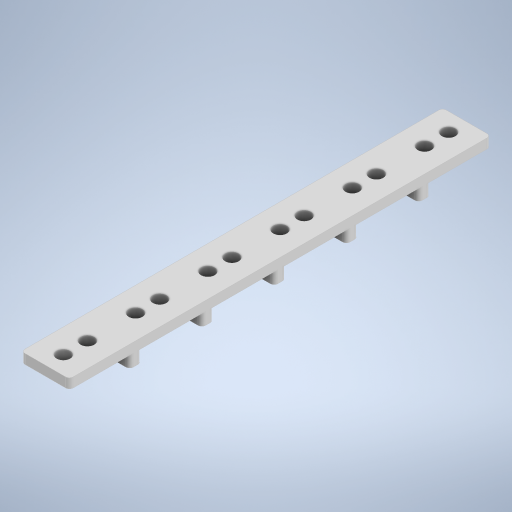
# Autodesk Inventor part: belka_poprzeg
Saved by Autodesk Inventor 2024.2 (Build 282272000, 272)
## iProperties
Created: 2024-01-12
Part Number: belka_poprzeg
Material: PLA
Document SubType Name: Modeling
Designer: Konrad
Density: 1 g/cm^3
Appearance: PLA
Author: Konrad
Autodesk Inventor part; units mm, degrees
ref_plane "YZ Plane" through (0, 0, 0) normal (1, 0, 0) x (0, 1, 0)
ref_plane "XZ Plane" through (0, 0, 0) normal (0, 1, 0) x (-1, 0, 0)
ref_plane "XY Plane" through (0, 0, 0) normal (0, 0, 1) x (1, 0, 0)
sketch "Szkic1" plane through (0, 0, 0) normal (0, 1, 0) x (-1, 0, 0)
  line L0 (0, 0) -> (20, 0)
  line L1 (20, 0) -> (20, -25)
  line L2 (20, -25) -> (0, -25)
  line L3 (0, -25) -> (0, 0)
  line L4 (0, -25) -> (20, -25)
  line L5 (20, -25) -> (20, -30)
  line L6 (20, -30) -> (0, -30)
  line L7 (0, -30) -> (0, -25)
  line L8 (0, -30) -> (20, -30)
  line L9 (0, -30) -> (20, -30)
  line L10 (20, -30) -> (20, -55)
  line L11 (20, -55) -> (0, -55)
  line L12 (0, -55) -> (0, -30)
  line L13 (0, -55) -> (20, -55)
  line L14 (20, -55) -> (20, -60)
  line L15 (20, -60) -> (0, -60)
  line L16 (0, -60) -> (0, -55)
  line L17 (0, -60) -> (12.1994, -60)
  line L18 (0, -60) -> (20, -60)
  line L19 (20, -60) -> (20, -85)
  line L20 (20, -85) -> (0, -85)
  line L21 (0, -85) -> (0, -60)
  line L22 (0, -85) -> (20, -85)
  line L23 (20, -85) -> (20, -90)
  line L24 (20, -90) -> (0, -90)
  line L25 (0, -90) -> (0, -85)
  line L26 (0, -90) -> (12.1994, -90)
  line L27 (0, -90) -> (20, -90)
  line L28 (20, -90) -> (20, -115)
  line L29 (20, -115) -> (0, -115)
  line L30 (0, -115) -> (0, -90)
  line L31 (0, -115) -> (20, -115)
  line L32 (20, -115) -> (20, -120)
  line L33 (20, -120) -> (0, -120)
  line L34 (0, -120) -> (0, -115)
  line L35 (0, -120) -> (3.8166, -120)
  line L36 (20, -120) -> (0, -120)
  line L37 (0, -120) -> (0, -145)
  line L38 (0, -145) -> (20, -145)
  line L39 (20, -145) -> (20, -120)
  circle A0 centre (10, -7.5) radius 2.8
  circle A1 centre (10, -17.5) radius 2.8
  line L40 (20, -42.5) -> (0, -42.5) construction
  line L41 (20, -72.5) -> (0, -72.5) construction
  line L42 (20, -102.5) -> (0, -102.5) construction
  line L43 (20, -132.5) -> (0, -132.5) construction
  line L44 (20, -12.5) -> (0, -12.5) construction
  circle A2 centre (10, -47.5) radius 2.8
  circle A3 centre (10, -37.5) radius 2.8
  circle A4 centre (10, -77.5) radius 2.8
  circle A5 centre (10, -67.5) radius 2.8
  circle A6 centre (10, -107.5) radius 2.8
  circle A7 centre (10, -97.5) radius 2.8
  circle A8 centre (10, -137.5) radius 2.8
  circle A9 centre (10, -127.5) radius 2.8
  circle A10 centre (10, -167.5) radius 2.8
  circle A11 centre (10, -157.5) radius 2.8
  line L45 (20, -145) -> (0, -145)
  line L46 (0, -145) -> (0, -150)
  line L47 (0, -150) -> (20, -150)
  line L48 (20, -150) -> (20, -145)
  line L49 (20, -150) -> (0, -150)
  line L50 (0, -150) -> (0, -175)
  line L51 (0, -175) -> (20, -175)
  line L52 (20, -175) -> (20, -150)
  line L53 (20, -162.5) -> (0, -162.5) construction
  dimension "d2" = 20
  dimension "d3" = 25
  dimension "d4" = 5
  dimension "d14" = 10
  dimension "d16" = 10
  dimension "d17" = 5.6
  dimension "d20" = 30
  constraints: 108 end point, 22 parallel, 15 horizontal, 12 centre point, 12 midpoint, 11 equal length, 11 perpendicular, 5 point on line, 1 equal radius, 1 symmetric about line, 1 vertical, 20 other
  measures "d2" distance of L0.start L0.end
  measures "d3" distance of L0.end L1.end
  measures "d4" distance of L4.end L5.end
  measures "d14" distance of A1.centre A0.centre
  measures "d16" distance from line of L3 A0.centre
  measures "d17" diameter of A0
  measures "d20" distance of A1.centre A2.centre
extrude "Wyciągnięcie proste1" add sketch "Szkic1" along normal blind 4
extrude "Wyciągnięcie proste2" add sketch "Szkic1" against normal blind 5 contours L2 L5 L6 L7 | L11 L14 L15 L16 | L20 L23 L24 L25 | L29 L32 L33 L34 | L38 L48 L47 L46
fillet "Zaokrąglenie1" radius 1.6 24 edges at (0, 2, 0) (-20, 2, 0) (0, 2, -175) (-20, 2, -175) (-20, -2.5, -150) (0, -2.5, -150) (0, -2.5, -145) (-20, -2.5, -145) (0, -2.5, -120) (0, -2.5, -115) (-20, -2.5, -120) (-20, -2.5, -115) (-20, -2.5, -90) (-20, -2.5, -85) (0, -2.5, -90) (0, -2.5, -85) (0, -2.5, -60) (0, -2.5, -55) (-20, -2.5, -55) (-20, -2.5, -60) (-20, -2.5, -30) (-20, -2.5, -25) (0, -2.5, -25) (0, -2.5, -30)
equation "\"d16\" = 0.5 * d2"
